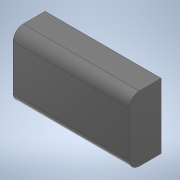
# Autodesk Inventor part: BH321-1P24
Saved by Autodesk Inventor 2022 (Build 260153000, 153)
## iProperties
Created: 2024-05-30
Part Number: BH321-1P24
Material: 一般
Document SubType Name: Modeling
Designer: yamashita1
Density: 1 g/cm^3
Appearance: 既定
Author: yamashita1
Autodesk Inventor part; units mm, degrees
ref_plane "YZ Plane" through (0, 0, 0) normal (1, 0, 0) x (0, 1, 0)
ref_plane "XZ Plane" through (0, 0, 0) normal (0, 1, 0) x (-1, 0, 0)
ref_plane "XY Plane" through (0, 0, 0) normal (0, 0, 1) x (1, 0, 0)
sketch "スケッチ1" plane through (0, 0, 0) normal (0, 0, 1) x (1, 0, 0)
  line L0 (-28.5, 16) -> (28.5, 16)
  line L1 (28.5, 16) -> (28.5, -16)
  line L2 (28.5, -16) -> (-28.5, -16)
  line L3 (-28.5, -16) -> (-28.5, 16)
  point P0 (0, 0)
  point P1 (-28.5, 0)
  point P2 (0, 16)
  dimension "d0" = 57
  dimension "d1" = 32
  constraints: 8 end point, 2 midpoint, 2 parallel, 1 horizontal, 1 horizontal alignment, 1 perpendicular, 1 vertical alignment
  measures "d0" distance of L1.end L2.end
  measures "d1" distance of L0.end L1.end
extrude "押し出し1" add sketch "スケッチ1" along normal blind 15.7
fillet "フィレット1" radius 5 2 edges at (0, 16, 15.7) (0, -16, 15.7)
sketch "スケッチ2" plane through (0, 0, 0) normal (0, 0, -1) x (-1, 0, 0)
  line L0 (26, 20.4284) -> (26, -20.6337) construction
  line L1 (0, 0) -> (36.4083, 0) construction
  line L2 (28.5, 16) -> (28.5, -16) construction
  circle A0 centre (26, 6.5) radius 0.4
  circle A1 centre (26, -6.5) radius 0.4
  dimension "d5" = 2.5
  dimension "d6" = 0.8
  dimension "d7" = 13
  constraints: 4 end point, 2 centre point, 2 point on line, 1 equal radius, 1 horizontal, 1 symmetric about line, 1 vertical
  measures "d5" distance between parallel lines of L2 L0
  measures "d6" diameter of A0
  measures "d7" distance of A1.centre A0.centre
extrude "押し出し2" add sketch "スケッチ2" along normal blind 2.8
